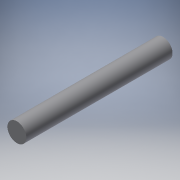
# Autodesk Inventor part: knapp
Saved by Autodesk Inventor 2019 (Build 230136000, 136)
## iProperties
Created: 2018-12-15
Part Number: knapp
Material: Generic
Document SubType Name: Modeling
Designer: Filip
Density: 1 g/cm^3
Appearance: Default
Author: Filip
Autodesk Inventor part; units mm, degrees
ref_plane "YZ Plane" through (0, 0, 0) normal (1, 0, 0) x (0, 1, 0)
ref_plane "XZ Plane" through (0, 0, 0) normal (0, 1, 0) x (-1, 0, 0)
ref_plane "XY Plane" through (0, 0, 0) normal (0, 0, 1) x (1, 0, 0)
sketch "Sketch1" plane through (0, 0, 0) normal (0, 0, 1) x (1, 0, 0)
  ellipse E0 centre (-11.1277, -68.1652) end of major axis (-11.1277, -66.4152) minor radius 1.7499
  point P0 (0, 0)
  constraints: 2 other
extrude "Extrusion1" add sketch "Sketch1" along normal mid plane 24
thicken "Thicken1" operation add thickness 3 both sides no extend neighbours yes toward (0, 0, 1) faces at (-11.7054, -68.0995, 12)
body "Solid1"
